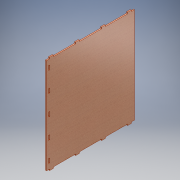
# Autodesk Inventor part: Fundo
Saved by Autodesk Inventor 2017 (Build 210142000, 142)
## iProperties
Created: 2017-10-02
Part Number: Fundo
Material: Wood (Oak)
Document SubType Name: Modeling
Designer: Felipe
Density: 0.76 g/cm^3
Appearance: White Oak - Natural Medium Gloss
Author: Felipe
Autodesk Inventor part; units mm, degrees
ref_plane "YZ Plane" through (0, 0, 0) normal (1, 0, 0) x (0, 1, 0)
ref_plane "XZ Plane" through (0, 0, 0) normal (0, 1, 0) x (-1, 0, 0)
ref_plane "XY Plane" through (0, 0, 0) normal (0, 0, 1) x (1, 0, 0)
sketch "Sketch1" plane through (0, 0, 0) normal (1, 0, 0) x (0, 1, 0)
  line L0 (0, 0) -> (830, 0) construction
  line L1 (830, 0) -> (830, -900)
  line L2 (830, -900) -> (0, -900) construction
  line L3 (0, -900) -> (0, 0)
  line L4 (800, 0) -> (765, 0) construction
  line L5 (765, 0) -> (765, 12.6635)
  line L6 (765, 12.6635) -> (800, 12.6635)
  line L7 (800, 12.6635) -> (800, 0)
  line L8 (555, 0) -> (520, 0) construction
  line L9 (520, 0) -> (520, 12.6635)
  line L10 (520, 12.6635) -> (555, 12.6635)
  line L11 (555, 12.6635) -> (555, 0)
  line L12 (310, 0) -> (275, 0) construction
  line L13 (275, 0) -> (275, 12.6635)
  line L14 (275, 12.6635) -> (310, 12.6635)
  line L15 (310, 12.6635) -> (310, 0)
  line L16 (65, 0) -> (30, 0) construction
  line L17 (30, 0) -> (30, 12.6635)
  line L18 (30, 12.6635) -> (65, 12.6635)
  line L19 (65, 12.6635) -> (65, 0)
  line L20 (830, -450) -> (0, -450) construction
  line L21 (800, -900) -> (765, -900) construction
  line L22 (765, -900) -> (765, -912.6635)
  line L23 (765, -912.6635) -> (800, -912.6635)
  line L24 (800, -912.6635) -> (800, -900)
  line L25 (555, -900) -> (520, -900) construction
  line L26 (520, -900) -> (520, -912.6635)
  line L27 (520, -912.6635) -> (555, -912.6635)
  line L28 (555, -912.6635) -> (555, -900)
  line L29 (310, -900) -> (275, -900) construction
  line L30 (275, -900) -> (275, -912.6635)
  line L31 (275, -912.6635) -> (310, -912.6635)
  line L32 (310, -912.6635) -> (310, -900)
  line L33 (65, -900) -> (30, -900) construction
  line L34 (30, -900) -> (30, -912.6635)
  line L35 (30, -912.6635) -> (65, -912.6635)
  line L36 (65, -912.6635) -> (65, -900)
  line L37 (830, -900) -> (800, -900)
  line L38 (765, -900) -> (555, -900)
  line L39 (520, -900) -> (310, -900)
  line L40 (275, -900) -> (65, -900)
  line L41 (30, -900) -> (0, -900)
  line L42 (830, 0) -> (800, 0)
  line L43 (765, 0) -> (555, 0)
  line L44 (520, 0) -> (310, 0)
  line L45 (275, 0) -> (65, 0)
  line L46 (30, 0) -> (0, 0)
  line L47 (20, -50) -> (30, -50)
  line L48 (30, -50) -> (30, -90)
  line L49 (30, -90) -> (20, -90)
  line L50 (20, -90) -> (20, -50)
  line L51 (20, -240) -> (30, -240)
  line L52 (30, -240) -> (30, -280)
  line L53 (30, -280) -> (20, -280)
  line L54 (20, -280) -> (20, -240)
  line L55 (20, -430) -> (30, -430)
  line L56 (30, -430) -> (30, -470)
  line L57 (30, -470) -> (20, -470)
  line L58 (20, -470) -> (20, -430)
  line L59 (20, -620) -> (30, -620)
  line L60 (30, -620) -> (30, -660)
  line L61 (30, -660) -> (20, -660)
  line L62 (20, -660) -> (20, -620)
  line L63 (20, -810) -> (30, -810)
  line L64 (30, -810) -> (30, -850)
  line L65 (30, -850) -> (20, -850)
  line L66 (20, -850) -> (20, -810)
  dimension "d0" = 900
  dimension "d1" = 830
  dimension "d2" = 35
  dimension "d3" = 30
  dimension "d4" = 210
  dimension "d5" = 210
  dimension "d6" = 210
  dimension "d7" = 30
  dimension "d11" = 40
  dimension "d12" = 10
  dimension "d15" = 40
  dimension "d16" = 10
  dimension "d17" = 40
  dimension "d18" = 10
  dimension "d19" = 40
  dimension "d20" = 10
  dimension "d21" = 40
  dimension "d22" = 10
  dimension "d23" = 150
  dimension "d24" = 150
  dimension "d25" = 150
  dimension "d26" = 150
  dimension "d27" = 50
  dimension "d28" = 50
  dimension "d31" = 20
  constraints: 134 end point, 20 parallel, 16 symmetric about line, 11 perpendicular, 10 horizontal, 9 collinear, 8 point on line, 4 equal length, 2 midpoint
  measures "d0" distance of L0.end L1.end
  measures "d1" distance of L0.start L0.end
  measures "d2" distance of L5.end L6.end
  measures "d3" distance between parallel lines of L3 L17
  measures "d4" distance between parallel lines of L19 L13
  measures "d5" distance between parallel lines of L9 L15
  measures "d6" distance between parallel lines of L5 L11
  measures "d7" distance between parallel lines of L1 L7
  measures "d11" distance of L47.end L48.end
  measures "d12" distance of L47.start L47.end
  measures "d15" distance of L52.start L52.end
  measures "d16" distance of L54.end L52.start
  measures "d17" distance of L56.start L56.end
  measures "d18" distance of L58.end L56.start
  measures "d19" distance of L60.start L60.end
  measures "d20" distance of L62.end L60.start
  measures "d21" distance of L64.start L64.end
  measures "d22" distance of L66.end L64.start
  measures "d23" distance between parallel lines of L51 L49
  measures "d24" distance between parallel lines of L53 L55
  measures "d25" distance between parallel lines of L57 L59
  measures "d26" distance between parallel lines of L63 L61
  measures "d27" distance between parallel lines of L46 L47
  measures "d28" distance between parallel lines of L2 L65
  measures "d31" distance between parallel lines of L3 L54
extrude "Extrusion3" add sketch "Sketch1" along normal blind 10
body "Solid3"
